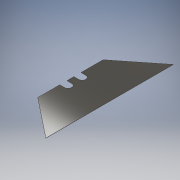
# Autodesk Inventor part: blade
Saved by Autodesk Inventor 2019 (Build 230136000, 136)
## iProperties
Created: 2019-03-02
Part Number: blade
Material: Stainless Steel
Document SubType Name: Modeling
Designer: assman
Density: 8 g/cm^3
Appearance: Steel - Polished
Author: assman
Autodesk Inventor part; units mm, degrees
ref_plane "YZ Plane" through (0, 0, 0) normal (1, 0, 0) x (0, 1, 0)
ref_plane "XZ Plane" through (0, 0, 0) normal (0, 1, 0) x (-1, 0, 0)
ref_plane "XY Plane" through (0, 0, 0) normal (0, 0, 1) x (1, 0, 0)
sketch "Sketch1" plane through (0, 0, 0) normal (0, 1, 0) x (-1, 0, 0)
  line L0 (11.093, 15.75) -> (42.593, 15.75) construction
  line L1 (-7.807, 30.75) -> (-7.807, -30.75)
  line L2 (11.093, 15.75) -> (-7.807, 30.75)
  line L3 (11.093, -15.75) -> (-7.807, -30.75)
  line L4 (11.093, 15.75) -> (11.093, 5.15) construction
  line L5 (11.093, -15.75) -> (11.093, -5.15) construction
  line L6 (11.093, 5.15) -> (8.843, 5.15)
  line L7 (8.843, 1.65) -> (11.093, 1.65)
  line L8 (11.093, -5.15) -> (8.843, -5.15)
  line L9 (8.843, -1.65) -> (11.093, -1.65)
  line L10 (11.093, 15.75) -> (11.093, 5.15)
  line L11 (11.093, 1.65) -> (11.093, -1.65)
  line L12 (11.093, -5.15) -> (11.093, -15.75)
  arc A0 (8.843, -1.65) -> (8.843, -5.15) centre (8.843, -3.4) ccw
  arc A1 (8.843, 5.15) -> (8.843, 1.65) centre (8.843, 3.4) ccw
  point P0 (0, 0)
  point P1 (-7.807, 0)
  point P2 (11.093, 0)
  dimension "d0" = 31.5
  dimension "d2" = 61.5
  dimension "d4" = 10.6
  dimension "d5" = 10.6
  dimension "d9" = 3.5
  dimension "d10" = 3.5
  dimension "d11" = 4
  dimension "d12" = 4
  constraints: 26 end point, 6 perpendicular, 4 point on circle, 4 tangent, 4 vertical, 3 horizontal, 2 centre point, 2 midpoint
  measures "d0" distance of L0.start L3.start
  measures "d2" distance of L1.start L1.end
  measures "d4" distance of L0.start L4.end
  measures "d5" distance of L3.start L5.end
  measures "d9" distance between parallel lines of L8 L9
  measures "d10" distance between parallel lines of L7 L6
extrude "Extrusion1" add sketch "Sketch1" along normal blind 0.1
body "Solid1"
